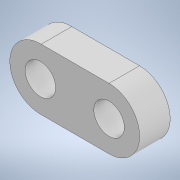
# Autodesk Inventor part: Lacznik
Saved by Autodesk Inventor 2021 (Build 250183000, 183)
## iProperties
Created: 2020-04-12
Part Number: Lacznik
Material: Ogólny
Document SubType Name: Modeling
Designer: dyrag
Density: 1 g/cm^3
Appearance: Domyślna
Author: dyrag
Autodesk Inventor part; units mm, degrees
ref_plane "YZ Plane" through (0, 0, 0) normal (1, 0, 0) x (0, 1, 0)
ref_plane "XZ Plane" through (0, 0, 0) normal (0, 1, 0) x (-1, 0, 0)
ref_plane "XY Plane" through (0, 0, 0) normal (0, 0, 1) x (1, 0, 0)
sketch "Szkic1" plane through (0, 0, 0) normal (0, 0, 1) x (1, 0, 0)
  line L0 (0.3069, -8.009) -> (9, -8.009)
  line L1 (0.3069, 7.997) -> (-8.7813, 7.997)
  line L2 (0.3069, -8.009) -> (-9.2187, -8.003)
  line L3 (0.3069, 7.997) -> (8.994, 7.997)
  circle A0 centre (9, -0.006) radius 4
  circle A1 centre (-9, -0.003) radius 4
  arc A2 (9, -8.009) -> (8.994, 7.997) centre (9, -0.006) ccw
  arc A3 (-8.7813, 7.997) -> (-9.2187, -8.003) centre (-9, -0.003) ccw
  point P0 (0, 0)
  dimension "d2" = 18
  dimension "d5" = 16
  dimension "d6" = 8
  constraints: 8 end point, 4 centre point, 4 point on circle, 2 coincident, 2 horizontal
  measures "d2" distance of A0.centre A1.centre
  measures "d5" vertical distance of L2.end L1.end
  measures "d6" diameter of A1
extrude "Wyciągnięcie proste1" add sketch "Szkic1" along normal blind 8
